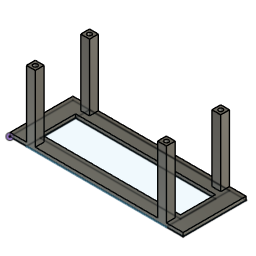
support ecran v1 (Autodesk Fusion 360 design; units mm, degrees)
Autodesk Fusion 360 part; units mm, degrees
sketch "Esquisse1" plane through (0, 0, 0) normal (0, 0, 1) x (1, 0, 0)
  line L0 (0, 0) -> (99, 0)
  line L1 (99, 0) -> (99, 36)
  line L2 (99, 36) -> (0, 36)
  line L3 (0, 36) -> (0, 0)
  line L4 (9.5, 36) -> (89.5, 36)
  line L5 (89.5, 36) -> (89.5, 0)
  line L6 (89.5, 0) -> (9.5, 0)
  line L7 (9.5, 0) -> (9.5, 36)
  line L8 (9.5, 8) -> (89.5, 8)
  line L9 (89.5, 8) -> (89.5, 28)
  line L10 (89.5, 28) -> (9.5, 28)
  line L11 (9.5, 28) -> (9.5, 8)
  dimension "d1" = 99
  dimension "d2" = 36
  dimension "d3" = 80
  dimension "d4" = 9.5
  dimension "d5" = 9.5
  dimension "d18" = 8
  dimension "d19" = 8
  constraint horizontal L0
  constraint vertical L1
  constraint horizontal L2
  constraint vertical L3
  constraint coincident L0.start L3.end
  constraint horizontal L4
  constraint vertical L5
  constraint horizontal L6
  constraint vertical L7
  constraint coincident L2 L4.start
  constraint horizontal L8
  constraint vertical L9
  constraint horizontal L10
  constraint vertical L11
  constraint coincident L5 L9.end
  constraint coincident L7 L8.start
  measures "d1" distance of L0.start L0.end
  measures "d2" distance of L0.start L2.end
  measures "d3" distance of L4.start L4.end
  measures "d4" distance of L3 L7
  measures "d5" distance of L1 L5
  measures "d18" distance of L4 L10
  measures "d19" distance of L0 L8
extrude "Extrusion1" add sketch "Esquisse1" along normal blind 2 contours L0 L2 L3 L7 L11 | L0 L5 L6 L7 L8 | L0 L1 L2 L5 L9 | L2 L4 L5 L7 L10
sketch "Esquisse2" plane through (0, 0, 2) normal (0, 0, 1) x (-1, 0, 0)
  line L0 (-99, 0) -> (-99, -36)
  line L1 (-99, -36) -> (0, -36)
  line L2 (0, -36) -> (0, 0)
  line L3 (0, 0) -> (-99, 0)
  line L4 (-9.5, -36) -> (-14.5, -36)
  line L5 (-14.5, -36) -> (-14.5, -31)
  line L6 (-14.5, -31) -> (-9.5, -31)
  line L7 (-9.5, -31) -> (-9.5, -36)
  line L8 (-89.5, -36) -> (-84.5, -36)
  line L9 (-84.5, -36) -> (-84.5, -31)
  line L10 (-84.5, -31) -> (-89.5, -31)
  line L11 (-89.5, -31) -> (-89.5, -36)
  line L12 (-89.4436, 0) -> (-84.4436, 0)
  line L13 (-84.4436, 0) -> (-84.4436, -5)
  line L14 (-84.4436, -5) -> (-89.4436, -5)
  line L15 (-89.4436, -5) -> (-89.4436, 0)
  line L16 (-9.5, 0) -> (-14.5, 0)
  line L17 (-14.5, 0) -> (-14.5, -5)
  line L18 (-14.5, -5) -> (-9.5, -5)
  line L19 (-9.5, -5) -> (-9.5, 0)
  line L20 (-9.5, -8) -> (-9.5, -28)
  line L21 (-9.5, -28) -> (-89.5, -28)
  line L22 (-89.5, -28) -> (-89.5, -8)
  line L23 (-89.5, -8) -> (-9.5, -8)
  dimension "d8" = 5
  dimension "d9" = 5
  dimension "d10" = 5
  dimension "d11" = 5
  dimension "d12" = 5
  dimension "d13" = 5
  dimension "d14" = 5
  dimension "d15" = 5
  constraint horizontal L4
  constraint vertical L5
  constraint horizontal L6
  constraint vertical L7
  constraint coincident L1 L4.start
  constraint horizontal L8
  constraint vertical L9
  constraint horizontal L10
  constraint vertical L11
  constraint coincident L1 L8.start
  constraint horizontal L12
  constraint vertical L13
  constraint horizontal L14
  constraint vertical L15
  constraint coincident L3 L12.start
  constraint horizontal L16
  constraint vertical L17
  constraint horizontal L18
  constraint vertical L19
  constraint coincident L3 L16.start
  measures "d8" distance of L4.start L4.end
  measures "d9" distance of L4.start L6.end
  measures "d10" distance of L8.start L8.end
  measures "d11" distance of L8.start L10.end
  measures "d12" distance of L12.start L12.end
  measures "d13" distance of L12.start L14.end
  measures "d14" distance of L16.start L16.end
  measures "d15" distance of L16.start L18.end
extrude "Extrusion2" add sketch "Esquisse2" along normal blind 38 contours L3 L12 L13 L14 L15 | L1 L8 L9 L10 L11 | L3 L16 L17 L18 L19 | L1 L4 L5 L6 L7
sketch "Esquisse3" plane through (0, 0, 40) normal (0, 0, 1) x (-1, 0, 0)
  line L0 (-9.5, -31) -> (-14.5, -31)
  line L1 (-14.5, -31) -> (-14.5, -36)
  line L2 (-14.5, -36) -> (-9.5, -36)
  line L3 (-9.5, -36) -> (-9.5, -31)
  circle A0 centre (-12, -33.5) radius 1.25
  circle A1 centre (-12, -2.5) radius 1.25
  line L4 (-14.5, -5) -> (-9.5, -5)
  line L5 (-9.5, 0) -> (-9.5, -36)
  circle A2 centre (-87, -33.5) radius 1.25
  line L6 (-99, -36) -> (0, -36)
  line L7 (-89.5, -36) -> (-89.5, 0)
  circle A3 centre (-87, -2.5) radius 1.25
  line L8 (-89.5, 0) -> (-9.5, 0)
  dimension "d20" = 2.5
  dimension "d21" = 2.5
  dimension "d22" = 2.5
  dimension "d23" = 2.5
  dimension "d24" = 2.5
  dimension "d25" = 2.5
  dimension "d26" = 2.5
  dimension "d27" = 2.5
  dimension "d28" = 2.5
  dimension "d29" = 2.5
  dimension "d30" = 2.5
  dimension "d31" = 2.5
  measures "d20" diameter of A0
  measures "d21" diameter of A1
  measures "d22" distance of A1.centre L4
  measures "d23" distance of A1.centre L5
  measures "d24" distance of A0.centre L5
  measures "d25" distance of L0 A0.centre
  measures "d26" diameter of A2
  measures "d27" distance of A2.centre L6
  measures "d28" distance of A2.centre L7
  measures "d29" diameter of A3
  measures "d30" distance of L7 A3.centre
  measures "d31" distance of A3.centre L8
extrude "Extrusion3" cut sketch "Esquisse3" against normal blind 3 contours A0 | A1 | A2 | A3
